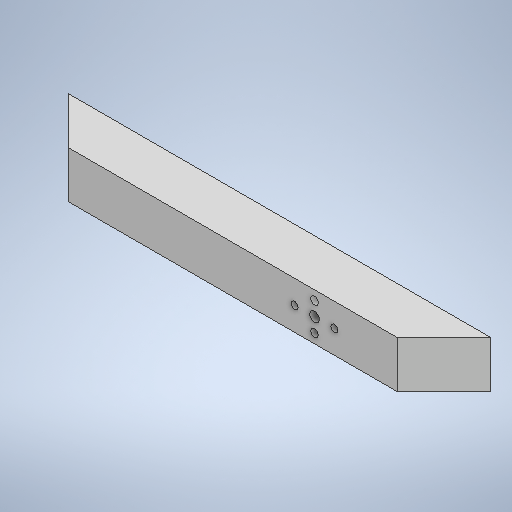
# Autodesk Inventor part: TS_Positionierungseinheit_Rahmen_int
Saved by Autodesk Inventor 2025.1 (Build 291241000, 241)
## iProperties
Created: 2025-05-23
Part Number: TS_Positionierungseinheit_Rahmen_int
Material: Generisch
Document SubType Name: Modeling
Designer: tino
Density: 1 g/cm^3
Appearance: Vorgabe
Author: tino
Autodesk Inventor part; units mm, degrees
ref_plane "XZ Plane" through (0, 0, 0) normal (0, 1, 0) x (-1, 0, 0)
ref_plane "XY Plane" through (0, 0, 0) normal (0, 0, 1) x (1, 0, 0)
sketch "Skizze1" plane through (0, 0, 0) normal (0, 1, 0) x (-1, 0, 0)
  line L0 (180.5, 20) -> (-180.5, 20)
  line L1 (-180.5, 20) -> (-180.5, -20)
  line L2 (-180.5, -20) -> (180.5, -20)
  line L3 (180.5, -20) -> (180.5, 20)
  line L4 (180.5, 20) -> (-180.5, -20) construction
  line L5 (-180.5, 20) -> (180.5, -20) construction
  point P0 (0, 0)
  dimension "d0" = 361
  dimension "d1" = 40
  constraints: 12 end point, 2 midpoint, 2 parallel, 1 horizontal, 1 perpendicular
  measures "d0" distance of L0.start L0.end
  measures "d1" distance of L2.end L0.start
extrude "Extrusion1" add sketch "Skizze1" along normal mid plane 40
chamfer "Fasen1" distance 40 angle 45 2 edges at (-180.5, -20, 0) (180.5, -20, 0)
sketch "Skizze2" plane through (0, 20, 0) normal (0, 1, 0) x (1, 0, 0)
  line L0 (180.5, -20) -> (180.5, 20) projected
  line L1 (-180.5, 20) -> (-180.5, -20) projected
  line L2 (180.5, 20) -> (-180.5, 20) projected
  line L3 (-180.5, 0) -> (180.5, 0) construction
  line L4 (-180.5, -20) -> (180.5, -20) projected
  line L5 (70, -20) -> (70, 20) construction
  point P0 (0, 0)
  point P1 (70, 0)
  point P2 (87, 0)
  point P3 (53, 0)
  point P4 (70, -12)
  point P5 (70, 12)
  point P6 (70, 0)
  dimension "d24" = 20
  dimension "d25" = 17
  dimension "d26" = 17
  dimension "d34" = 70
  dimension "d35" = 12
  dimension "d36" = 12
  constraints: 7 point on line, 4 end point, 4 midpoint, 2 perpendicular
  measures "d24" distance between parallel lines of L2 L3
  measures "d25" distance of point (70, 0) point (53, 0)
  measures "d26" distance of point (87, 0) point (70, 0)
  measures "d34" distance from line of point (0, 0) L5
  measures "d35" distance of point (70, 0) point (70, 12)
  measures "d36" distance of point (70, -12) point (70, 0)
hole "Bohrung1" at (87, 20, 0) at (53, 20, 0) direction (0, -1, 0) diameter 6 end through all
hole "Hole3" at (70, 20, 0) direction (0, -1, 0) diameter 8.4 end through all counterbore diameter 15 counterbore depth 8.6
hole "Hole4" at (70, 20, 12) at (70, 20, -12) direction (0, -1, 0) diameter 6.647 end through all thread size "M8x1.25" class "6H" standard "ISO Metric profile"
ref_plane "Work Plane1" through (70, 20, 12) normal (1, 0, 0) x (0, 1, 0)
equation "\"d0\" = Laenge_Rahmen"
equation "\"d1\" = Breite_Rahmen"
equation "\"d2\" = Hoehe_Rahmen"
equation "\"d4\" = Breite_Rahmen"
equation "\"d24\" = Abstand_Bohrung_Rahmen"
equation "\"d25\" = 0.5 * Abtand_Fuehrungsstifte"
equation "\"d26\" = d25"
equation "\"d34\" = Exzentrizität"
equation "\"d35\" = Madenschraube_Abstand"
equation "\"d36\" = d35"
equation "\"d9\" = Durchmesser_Stifte"
equation "\"Breite_Rahmen\" = 40"
equation "\"Hoehe_Rahmen\" = Breite_Rahmen"
equation "\"Breite_Bauteiltraeger\" = 239"
equation "\"Lange_Bauteiltraeger\" = Breite_Bauteiltraeger"
equation "\"Laenge_Rahmen\" = Innenmaß_Rahmen + 2 * Breite_Rahmen"
equation "\"Toleranz_Verstellung\" = 1"
equation "\"Abtand_Fuehrungsstifte\" = 34"
equation "\"Durchmesser_Stifte\" = 6"
equation "\"Abstand_Bohrung_Rahmen\" = 20"
equation "\"Exzentrizität\" = 70"
equation "\"Madenschraube_Abstand\" = 12"
equation "\"Innenmaß_Rahmen\" = 281"
